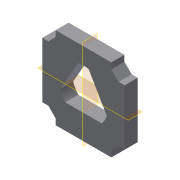
# Autodesk Inventor part: 20_IM_Cube_Insert_Lens_holder_RMS_63x
Saved by Autodesk Inventor 2019.4 (Build 234330000, 330)
## iProperties
Created: 2019-10-23
Part Number: 20_IM_Cube_Insert_Lens_holder_RMS_63x
Material: Generic
Document SubType Name: Modeling
Designer: marsikovabarbora
Density: 1 g/cm^3
Appearance: Default
Lens_diameter: 25,000 mm
Author: marsikovabarbora
Autodesk Inventor part; units mm, degrees
ref_plane "YZ Plane" through (0, 0, 0) normal (1, 0, 0) x (0, 1, 0)
ref_plane "XZ Plane" through (0, 0, 0) normal (0, 1, 0) x (-1, 0, 0)
ref_plane "XY Plane" through (0, 0, 0) normal (0, 0, 1) x (1, 0, 0)
sketch "Sketch1" plane through (0, 0, 0) normal (0, 0, 1) x (1, 0, 0)
  line L0 (-35.2109, 0) -> (35.2109, 0) construction
  line L1 (0, -35.2109) -> (0, 35.2109) construction
  line L2 (0, 0) -> (13.4339, 13.4339) construction
  line L3 (0, 0) -> (18.9985, 0) construction
  line L4 (0, 25.1006) -> (17, 25.1006)
  line L5 (17, 25.1006) -> (17, 21.4406)
  line L6 (17, 21.4406) -> (19.2203, 19.2203)
  line L7 (25.1006, 0) -> (25.1006, 17)
  line L8 (25.1006, 17) -> (21.4406, 17)
  line L9 (21.4406, 17) -> (19.2203, 19.2203)
  line L10 (0, 0) -> (-13.4339, 13.4339) construction
  line L11 (0, 0) -> (-18.9985, 0) construction
  line L12 (0, 25.1006) -> (-17, 25.1006)
  line L13 (-17, 25.1006) -> (-17, 21.4406)
  line L14 (-17, 21.4406) -> (-19.2203, 19.2203)
  line L15 (-25.1006, 0) -> (-25.1006, 17)
  line L16 (-25.1006, 17) -> (-21.4406, 17)
  line L17 (-21.4406, 17) -> (-19.2203, 19.2203)
  line L18 (0, 0) -> (13.4339, -13.4339) construction
  line L19 (0, -25.1006) -> (17, -25.1006)
  line L20 (17, -25.1006) -> (17, -21.4406)
  line L21 (17, -21.4406) -> (19.2203, -19.2203)
  line L22 (25.1006, 0) -> (25.1006, -17)
  line L23 (25.1006, -17) -> (21.4406, -17)
  line L24 (21.4406, -17) -> (19.2203, -19.2203)
  line L25 (0, 0) -> (-13.4339, -13.4339) construction
  line L26 (0, -25.1006) -> (-17, -25.1006)
  line L27 (-17, -25.1006) -> (-17, -21.4406)
  line L28 (-17, -21.4406) -> (-19.2203, -19.2203)
  line L29 (-25.1006, 0) -> (-25.1006, -17)
  line L30 (-25.1006, -17) -> (-21.4406, -17)
  line L31 (-21.4406, -17) -> (-19.2203, -19.2203)
  line L32 (-17.05, 25.1506) -> (0, 25.1506)
  line L33 (0, 25.1506) -> (17.05, 25.1506)
  line L34 (17.05, 25.1506) -> (17.05, 21.4613)
  line L35 (17.05, 21.4613) -> (19.2557, 19.2557)
  line L36 (19.2557, 19.2557) -> (21.4613, 17.05)
  line L37 (21.4613, 17.05) -> (25.1506, 17.05)
  line L38 (25.1506, 17.05) -> (25.1506, 0)
  line L39 (25.1506, 0) -> (25.1506, -17.05)
  line L40 (25.1506, -17.05) -> (21.4613, -17.05)
  line L41 (21.4613, -17.05) -> (19.2557, -19.2557)
  line L42 (19.2557, -19.2557) -> (17.05, -21.4613)
  line L43 (17.05, -21.4613) -> (17.05, -25.1506)
  line L44 (17.05, -25.1506) -> (0, -25.1506)
  line L45 (0, -25.1506) -> (-17.05, -25.1506)
  line L46 (-17.05, -25.1506) -> (-17.05, -21.4613)
  line L47 (-17.05, -21.4613) -> (-19.2557, -19.2557)
  line L48 (-19.2557, -19.2557) -> (-21.4613, -17.05)
  line L49 (-21.4613, -17.05) -> (-25.1506, -17.05)
  line L50 (-25.1506, -17.05) -> (-25.1506, 0)
  line L51 (-25.1506, 0) -> (-25.1506, 17.05)
  line L52 (-25.1506, 17.05) -> (-21.4613, 17.05)
  line L53 (-21.4613, 17.05) -> (-19.2557, 19.2557)
  line L54 (-19.2557, 19.2557) -> (-17.05, 21.4613)
  line L55 (-17.05, 21.4613) -> (-17.05, 25.1506)
  dimension "d0" = 45
  dimension "d1" = 3.14
  dimension "d2" = 3.66
  dimension "d3" = 17
  dimension "d23" = 0.05
  constraints: 108 end point, 24 symmetric about line, 5 point on line, 3 perpendicular, 2 horizontal, 1 equal length, 23 other
  measures "d0" angle of L3 L2
  measures "d1" distance of L5.end L6.end
  measures "d2" distance of L4.end L5.end
  measures "d3" distance of L4.start L4.end
  measures "d23" distance between parallel lines of L12 L32
extrude "Extrusion1" add sketch "Sketch1" along normal blind 8 contours L4 L5 L6 L9 L8 L7 L22 L23 L24 L21 L20 L19 L26 L27 L28 L31 L30 L29 L15 L16 L17 L14 L13 L12 | L32 L33 L34 L35 L36 L37 L38 L39 L40 L41 L42 L43 L44 L45 L46 L47 L48 L49 L50 L51 L52 L53 L54 L55
ref_plane "Work Plane1" through (0, -17.05, 0) normal (1, 0, 0) x (0, 0, -1)
ref_plane "Work Plane2" through (-17.05, 0, 0) normal (0, 1, 0) x (1, 0, 0)
sketch "Sketch4" plane through (0, 0, 8) normal (0, 0, 1) x (1, 0, 0)
  line L0 (-21.4613, 17.05) -> (-25.1506, 17.05) projected
  line L1 (17.05, 25.1506) -> (-17.05, 25.1506) projected
  line L2 (-17.05, 25.1506) -> (-17.05, 21.4613) projected
  line L3 (-17.05, 21.4613) -> (-21.4613, 17.05) projected
  line L4 (-21.4613, 17.05) -> (-25.1506, 17.05) projected
  line L5 (-25.1506, 17.05) -> (-25.1506, -17.05) projected
  line L6 (-25.1506, -17.05) -> (-21.4613, -17.05) projected
  line L7 (-21.4613, -17.05) -> (-17.05, -21.4613) projected
  line L8 (-17.05, -21.4613) -> (-17.05, -25.1506) projected
  line L9 (-17.05, -25.1506) -> (17.05, -25.1506) projected
  line L10 (17.05, -25.1506) -> (17.05, -21.4613) projected
  line L11 (17.05, -21.4613) -> (21.4613, -17.05) projected
  line L12 (21.4613, -17.05) -> (25.1506, -17.05) projected
  line L13 (25.1506, -17.05) -> (25.1506, 17.05) projected
  line L14 (25.1506, 17.05) -> (21.4613, 17.05) projected
  line L15 (21.4613, 17.05) -> (17.05, 21.4613) projected
  line L16 (17.05, 21.4613) -> (17.05, 25.1506) projected
  circle A0 centre (22.1506, 12) radius 1.45 projected
  circle A1 centre (22.1506, -12) radius 1.45 projected
  circle A2 centre (-1.8494, -12) radius 1.45 projected
  circle A3 centre (-1.8494, 12) radius 1.45 projected
  circle A4 centre (0, 0) radius 25.1506
  circle A5 centre (0, 0) radius 10
  point P0 (0, 0)
  dimension "d27" = 20
  constraints: 3 tangent, 2 centre point, 1 coincident
  measures "d27" diameter of A5
extrude "Extrusion4" cut sketch "Sketch4" against normal through all contours A4 A0 | A0 A4 | A4 A1 | A1 A4 | A2 | A3 | A5
equation "\"Lens_diameter\" = 25"
body "Solid1"
